# Autodesk Inventor part: Welle
Saved by Autodesk Inventor 2016 (Build 200138000, 138)
## iProperties
Created: 2015-09-09
Part Number: Welle
Material: Steel
Document SubType Name: Modeling
Designer: 4ndreas
Density: 7.85 g/cm^3
Appearance: Steel
Mass: 11.0627 g
Surface Area: 9.87334 cm^2
Volume: 1.40927 cm^3
CustomPartVersion: 1
Author: 4ndreas
Autodesk Inventor part; units mm, degrees
ref_plane "Startebene" through (0, 0, 0) normal (1, 0, 0) x (0, 1, 0)
ref_plane "XZ Plane" through (0, 0, 0) normal (0, 1, 0) x (-1, 0, 0)
ref_plane "XY Plane" through (0, 0, 0) normal (0, 0, 1) x (1, 0, 0)
sketch "Hauptskizze" plane through (0, 0, 0) normal (0, 0, 1) x (1, 0, 0)
  line L0 (0, 0) -> (50, 0)
  line L1 (0, 0) -> (0, 3)
  line L2 (50, 3) -> (50, 0)
  line L3 (0, 3) -> (50, 3)
  dimension "d3" = 6
  constraints: 8 end point, 2 vertical, 1 horizontal
  measures "d3" diameter of L3 L0
revolve "Umdrehung1" add sketch "Hauptskizze" angle 360 about axis through (0, 0, 0) along (1, 0, 0)
chamfer "Fase3" distance 0.5 angle 45 1 edges at (0, -3, 0) measured on face at (33.3333, 2.9612, -0.4812)
chamfer "Fase2" distance 0.5 angle 45 1 edges at (50, -3, 0) measured on face at (17, 2.9903, -0.2414)
